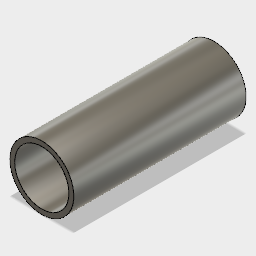
camera handle TAO part2 v2 (Autodesk Fusion 360 design; units mm, degrees)
Autodesk Fusion 360 part; units mm, degrees
sketch "Sketch1" plane through (0, 0, 0) normal (0, 0, 1) x (1, 0, 0)
  circle A0 centre (20, 20) radius 13
  dimension "d1" = 26
  measures "d1" diameter of A0
extrude "Extrude1" add sketch "Sketch1" along normal blind 70
sketch "Sketch2" plane through (0, 0, 70) normal (0, 0, 1) x (1, 0, 0)
  circle A0 centre (20, 20) radius 13
  circle A1 centre (20, 20) radius 11
  dimension "d4" = 2
extrude "Extrude2" cut sketch "Sketch2" against normal up to surface (70 mm away) contours A1
sketch "Sketch3" plane through (0, 0, 0) normal (1, 0, 0) x (0, 0, -1)
  line L0 (-50.7051, 17.6488) -> (-43.7051, 17.6488)
  line L1 (-43.7051, 17.6488) -> (-43.7051, 24.6488)
  line L2 (-43.7051, 24.6488) -> (-50.7051, 24.6488)
  line L3 (-50.7051, 24.6488) -> (-50.7051, 17.6488)
  line L4 (-50.7051, 17.6488) -> (-43.7051, 24.6488) construction
  line L5 (-43.7051, 17.6488) -> (-50.7051, 24.6488) construction
  point P0 (-47.2051, 21.1488)
  dimension "d7" = 7
  dimension "d8" = 7
  measures "d7" distance of L1.end L2.end
  measures "d8" distance of L0.end L1.end
extrude "Extrude4" cut sketch "Sketch3" along normal blind 15
extrude "Extrude3" cut sketch "Sketch3" along normal blind 12
